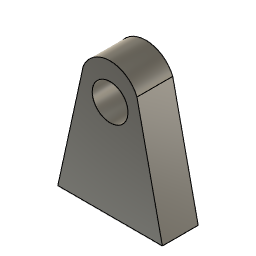
Main Shaft Support (Autodesk Fusion 360 design; units mm, degrees)
Autodesk Fusion 360 part; units mm, degrees
sketch "Sketch1" plane through (0, 0, 0) normal (0, 1, 0) x (1, 0, 0)
  circle A0 centre (0, 0) radius 1000
  arc A1 (-1500, -1000) -> (1500, -1000) centre (0, -375) ccw
  line L0 (-1500, -1000) -> (-2921.0842, 5496.3851)
  line L1 (0, -2600) -> (0, 5800) construction
  line L2 (1500, -1000) -> (2921.0842, 5496.3851)
  line L3 (-2921.0842, 5496.3851) -> (2921.0842, 5496.3851)
  constraint coincident A0.centre origin
  constraint vertical L1
  constraint symmetric A1.start L1 A1.end
  constraint symmetric L0.end L1 L2.end
extrude "Extrude1" add sketch "Sketch1" along normal blind 2000
